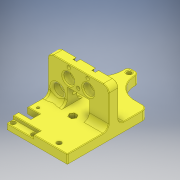
# Autodesk Inventor part: Extruder Mount cyclops mit ir probe _ rounded
Saved by Autodesk Inventor 2019 (Build 230136000, 136)
## iProperties
Created: 2016-03-27
Part Number: Extruder Mount cyclops mit ir probe _ rounded
Material: ABS Plastic
Document SubType Name: Modeling
Designer: Scott
Mass: 47.0424 g
Surface Area: 151.913 cm^2
Volume: 44.3796 cm^3
Density: 1.06 g/cm^3
Appearance: Smooth - Yellow
Author: Scott
## iProperties of the stored document Extruder Mount cyclops mit ir probe_3D-Druck.ipt
Created: 2018-12-29
Part Number: Extruder Mount cyclops mit ir probe_3D-Druck
Material: Generisch
Document SubType Name: Modeling
Designer: marc
Density: 1 g/cm^3
Appearance: Vorgabe
Author: marc
Autodesk Inventor part; units mm, degrees
ref_plane "YZ Plane" through (0, 0, 0) normal (1, 0, 0) x (0, 1, 0)
ref_plane "XZ Plane" through (0, 0, 0) normal (0, 1, 0) x (-1, 0, 0)
sketch "Sketch1" plane through (0, 0, 0) normal (0, 0, 1) x (1, 0, 0)
  line L0 (0, 0) -> (85, 0)
  line L1 (85, 0) -> (85, 83.5)
  line L2 (85, 83.5) -> (0, 83.5)
  line L3 (0, 83.5) -> (0, 0)
  dimension "d0" = 85
  dimension "d1" = 83.5
  constraints: 8 end point, 2 parallel, 1 horizontal, 1 perpendicular
  measures "d0" distance of L1.end L2.end
  measures "d1" distance of L0.end L1.end
extrude "Extrusion1" add sketch "Sketch1" along normal blind 5
sketch "Sketch10" plane through (0, 0, 5) normal (0, 0, 1) x (1, 0, 0)
  line L0 (85, 0) -> (85, 83.5) projected
  line L1 (85, 83.5) -> (0, 83.5) projected
  line L2 (0, 83.5) -> (0, 0) projected
  circle A0 centre (15.5, 75) radius 2.25 projected
  circle A1 centre (15.5, 75) radius 4
  circle A2 centre (33.5, 75) radius 4
  circle A3 centre (51.5, 75) radius 4
  circle A4 centre (69.5, 75) radius 4
  circle A5 centre (33.5, 51) radius 2.25 projected
  line L3 (0, 0) -> (85, 0) projected
  circle A6 centre (33.5, 30) radius 4
  circle A7 centre (51.5, 30) radius 4
  circle A8 centre (33.5, 6) radius 4
  circle A9 centre (51.5, 6) radius 4
  line L4 (85, 0) -> (85, 83.5) projected
  line L5 (85, 83.5) -> (0, 83.5) projected
  line L6 (0, 83.5) -> (0, 0) projected
  line L7 (0, 0) -> (85, 0) projected
  circle A10 centre (15.5, 51) radius 2.25 projected
  circle A11 centre (15.5, 51) radius 4
  circle A12 centre (33.5, 51) radius 4
  circle A13 centre (51.5, 51) radius 4
  circle A14 centre (69.5, 51) radius 4
  circle A15 centre (37.75, 40.5) radius 1.5 projected
  circle A16 centre (47.25, 40.5) radius 1.5 projected
  circle A17 centre (37.75, 40.5) radius 2.75
  circle A18 centre (47.25, 40.5) radius 2.75
  dimension "d73" = 8
  dimension "d152" = 5.5
  constraints: 14 centre point, 12 equal radius, 5 coincident
  measures "d73" diameter of A1
  measures "d152" diameter of A17
extrude "Grundplatte" add sketch "Sketch10" along normal blind 4 contours L3 L2 L1 L0 | A0 | A1 | A2 | A3 | A4 | A5 | A6 | A7 | A8 | A9 | A10 | A11 | A12 | A13 | A14 | A15 | A16 | A17 | A18
sketch "Sketch24" plane through (0, 0, 9) normal (0, 0, 1) x (1, 0, 0)
  line L0 (9.5, 63.9289) -> (9.5, 2) projected
  line L1 (75.5, 2) -> (75.5, 63.9289) projected
  line L2 (75.5, 63.9289) -> (75.5, 2) projected
  line L3 (9.5, 46.85) -> (75.5, 46.85)
  line L4 (75.5, 46.85) -> (75.5, 38.15)
  line L5 (75.5, 38.15) -> (9.5, 38.15)
  line L6 (9.5, 38.15) -> (9.5, 46.85)
  line L7 (0, 0) -> (85, 0) projected
  point P0 (11.5, 0)
  point P1 (73.5, 0)
  dimension "d173" = 8.7
  dimension "d174" = 38.15
  constraints: 8 end point, 2 parallel, 2 point on line, 1 horizontal, 1 perpendicular
  measures "d173" distance between parallel lines of L5 L3
  measures "d174" distance between parallel lines of L7 L5
extrude "Hotend_Brücke" add sketch "Sketch24" along normal blind 34
sketch "Sketch25" plane through (2, 83.5, 0) normal (0, 1, 0) x (1, 0, 0)
  line L0 (40.5, -18) -> (40.5, -43) construction
  line L1 (73.5, -43) -> (7.5, -43) construction
  line L2 (30.5, -9) -> (30.5, -24.2)
  line L3 (30.5, -24.2) -> (50.5, -24.2)
  line L4 (83, -9) -> (-2, -9) projected
  line L5 (50.5, -24.2) -> (50.5, -9)
  line L6 (50.5, -9) -> (30.5, -9)
  point P0 (-2, 0)
  point P1 (0, -9)
  dimension "d177" = 20
  dimension "d348" = 15.2
  constraints: 10 end point, 1 collinear, 1 midpoint, 1 perpendicular, 1 vertical
  measures "d177" distance of L2.end L3.end
  measures "d348" distance of L2.start L2.end
extrude "Luftdurchlass" cut sketch "Sketch25" against normal through all
sketch "Sketch39" plane through (32.5, 46.85, 24.2) normal (0, 1, 0) x (1, 0, 0)
  line L0 (0, 0) -> (0, 15.2) projected
  circle A0 centre (0, 7.6) radius 1.25
  point P0 (-32.5, 24.2)
  dimension "d263" = 2.5
  constraints: 1 centre point, 1 midpoint
  measures "d263" diameter of A0
extrude "Extrusion35" cut sketch "Sketch39" against normal blind 4
fillet "Fillet23" radius 1 1 edges at (31.25, 42.85, 16.6)
sketch "Sketch40" plane through (32.5, 46.85, 24.2) normal (0, 1, 0) x (1, 0, 0)
  line L0 (20, 15.2) -> (20, 0) projected
  line L1 (24, 7.35) -> (33, 7.35)
  line L2 (34, 8.35) -> (34, 8.6)
  line L3 (34, 8.6) -> (23, 8.6)
  line L4 (23, 8.6) -> (23, 8.35)
  arc A0 (23, 8.35) -> (24, 7.35) centre (24, 8.35) ccw
  arc A1 (33, 7.35) -> (34, 8.35) centre (33, 8.35) ccw
  line L5 (20, 0) -> (0, 0) projected
  point P0 (-32.5, 24.2)
  point P1 (23, 7.35)
  dimension "d267" = 1.25
  dimension "d268" = 3
  dimension "d269" = 14
  dimension "d270" = 1
  dimension "d332" = 8.6
  constraints: 8 end point, 4 point on circle, 4 tangent, 2 centre point, 2 parallel, 2 point on line, 1 equal radius, 1 horizontal, 1 perpendicular
  measures "d267" distance of L3.end point (23, 7.35)
  measures "d268" distance between parallel lines of L4 L0
  measures "d269" distance between parallel lines of L2 L0
  measures "d270" radius of A0
  measures "d332" distance between parallel lines of L5 L3
revolve "Revolution1" cut sketch "Sketch40" angle 180 about axis through (66.5, 46.85, 15.6) along (1, 0, 0)
sketch "Sketch45" plane through (0, 0, 9) normal (0, 0, 1) x (1, 0, 0)
  line L0 (85, 83.5) -> (0, 83.5) projected
  line L1 (75.5, 46.85) -> (75.5, 63.9289) projected
  arc A0 (76.9645, 67.4645) -> (75.5, 63.9289) centre (80.5, 63.9289) ccw projected
  line L2 (76.9645, 67.4645) -> (84.4142, 74.9142) projected
  arc A1 (84.4142, 74.9142) -> (85, 76.3284) centre (83, 76.3284) ccw projected
  line L3 (85, 0) -> (85, 83.5) projected
  arc A2 (85, 81.5) -> (83, 83.5) centre (83, 81.5) ccw projected
  line L4 (85, 83.5) -> (0, 83.5) projected
  line L5 (75.5, 63.5) -> (85, 63.5)
  line L6 (85, 63.5) -> (85, 83.5)
  line L7 (85, 83.5) -> (75.5, 83.5)
  line L8 (75.5, 83.5) -> (75.5, 63.5)
  point P0 (0, 0)
  point P1 (43, 83.5)
  point P2 (75.5, 58.85)
  point P3 (41, 83.5)
  point P4 (75.5, 56.85)
  point P5 (2, 83.5)
  dimension "d301" = 20
  constraints: 9 end point, 2 parallel, 1 collinear, 1 horizontal, 1 perpendicular, 1 point on line
  measures "d301" distance between parallel lines of L0 L5
extrude "Extrusion39" cut sketch "Sketch45" against normal through all
sketch "Sketch51" plane through (0, 0, 0) normal (0, 0, -1) x (-1, 0, 0)
  line L0 (-75.5, 46.85) -> (-75.5, 38.15) construction
  line L1 (-9.5, 38.15) -> (-9.5, 46.85) construction
  line L2 (-75.5, 42.5) -> (-9.5, 42.5) construction
  line L3 (-75.5, 83.5) -> (0, 83.5) projected
  line L4 (0, 0) -> (-85, 0) projected
  line L5 (-70, 83.5) -> (-85, 83.5)
  line L6 (-85, 83.5) -> (-85, 0)
  line L7 (-85, 0) -> (-70, 0)
  line L8 (-70, 0) -> (-70, 83.5)
  line L9 (-42.5, 100.2) -> (-42.5, -16.7) projected
  line L10 (-15, 83.5) -> (0, 83.5)
  line L11 (0, 83.5) -> (0, 0)
  line L12 (0, 0) -> (-15, 0)
  line L13 (-15, 0) -> (-15, 83.5)
  dimension "d349" = 27.5
  dimension "d350" = 27.5
  constraints: 18 end point, 4 parallel, 2 horizontal, 2 midpoint, 2 perpendicular, 2 point on line
  measures "d349" distance between parallel lines of L8 L9
  measures "d350" distance between parallel lines of L13 L9
extrude "Extrusion43" cut sketch "Sketch51" against normal through all contours L3 L8 L4 L6 L5 | L3 L11 L4 L13
sketch "Sketch52" plane through (0, 0, 0) normal (0, 0, -1) x (-1, 0, 0)
  line L0 (-15, 46.85) -> (-15, 38.15) construction
  line L1 (-70, 38.15) -> (-70, 46.85) construction
  line L2 (-42.5, 100.2) -> (-42.5, -16.7) construction
  line L3 (-70, 83.5) -> (-15, 83.5) construction
  line L4 (-70, 83.5) -> (-70, 0) construction
  line L5 (-15, 0) -> (-70, 0) construction
  line L6 (-15, 0) -> (-15, 83.5) construction
  line L7 (-70, 83.5) -> (-15, 83.5) construction
  line L8 (-15, 83.5) -> (-15, 46.85) projected
  line L9 (-70, 83.5) -> (-15, 83.5)
  line L10 (-15, 83.5) -> (-15, 65.75)
  line L11 (-15, 65.75) -> (-70, 65.75)
  line L12 (-70, 65.75) -> (-70, 83.5)
  line L13 (-70, 41.75) -> (-15, 41.75) construction
  line L14 (-15, 0) -> (-70, 0) projected
  line L15 (-15, 38.15) -> (-15, 0) projected
  line L16 (-70, 0) -> (-15, 0)
  line L17 (-15, 0) -> (-15, 0.75)
  line L18 (-15, 0.75) -> (-70, 0.75)
  line L19 (-70, 0.75) -> (-70, 0)
  point P0 (0, 0)
  dimension "d353" = 24
  dimension "d373" = 65
  constraints: 18 end point, 4 parallel, 2 horizontal, 2 midpoint, 2 perpendicular, 2 point on line
  measures "d353" distance between parallel lines of L11 L13
  measures "d373" distance between parallel lines of L18 L11
extrude "Extrusion44" cut sketch "Sketch52" against normal through all
sketch "Sketch55" plane through (0, 0, 0) normal (0, 0, -1) x (-1, 0, 0)
  line L0 (-15, 0.75) -> (-15, 65.75) projected
  line L1 (-15, 65.75) -> (-15, 46.85) projected
  line L2 (-15, 38.15) -> (-15, 0.75) projected
  line L3 (-26, 46.75) -> (-15, 46.75)
  line L4 (-15, 46.75) -> (-15, 11.75)
  line L5 (-15, 11.75) -> (-26, 11.75)
  line L6 (-26, 11.75) -> (-26, 46.75)
  point P0 (0, 0)
  dimension "d374" = 19
  dimension "d375" = 11
  dimension "d376" = 11
  constraints: 8 end point, 2 parallel, 1 horizontal, 1 perpendicular, 1 point on line
  measures "d374" distance from line of L0.end L3
  measures "d375" distance from line of L0.start L5
  measures "d376" distance of L3.start L3.end
extrude "Extrusion45" cut sketch "Sketch55" against normal blind 3.5
sketch "Sketch56" plane through (0, 0, 0) normal (0, 0, -1) x (-1, 0, 0)
  line L0 (-70, 65.75) -> (-15, 65.75) construction
  line L1 (-42.5, 65.75) -> (-42.5, 0.75) construction
  line L2 (-15, 0.75) -> (-70, 0.75) construction
  line L3 (-54.5, 45.25) -> (-30.5, 45.25) construction
  line L4 (-30.5, 45.25) -> (-30.5, 21.25) construction
  line L5 (-30.5, 21.25) -> (-54.5, 21.25) construction
  line L6 (-54.5, 21.25) -> (-54.5, 45.25) construction
  line L7 (-30.5, 45.25) -> (-54.5, 21.25) construction
  line L8 (-54.5, 45.25) -> (-30.5, 21.25) construction
  point P0 (0, 0)
  point P1 (-42.5, 33.25)
  dimension "d379" = 24
  dimension "d380" = 24
  constraints: 14 end point, 4 midpoint, 3 coincident, 2 parallel, 1 horizontal, 1 perpendicular, 1 point on line
  measures "d379" distance of L3.start L3.end
  measures "d380" distance of L3.end L4.end
hole "Hole14" at (42.5, 33.25, 0) at (54.5, 45.25, 0) at (54.5, 21.25, 0) at (30.5, 21.25, 0) at (30.5, 45.25, 0) direction (0, 0, 1) diameter 3 depth 8
sketch "Sketch57" plane through (0, 0, 0) normal (0, 0, -1) x (-1, 0, 0)
  circle A0 centre (-42.5, 33.25) radius 1.5 projected
  point P0 (0, 0)
  constraints: 1 coincident
hole "Hole15" at (42.5, 33.25, 0) direction (0, 0, 1) diameter 4.2 end through all
ref_plane "Work Plane14" through (42.5, 37.25, 33.75) normal (1, 0, 0) x (0, -1, 0)
sketch "Sketch58" plane through (0, 0, 3.5) normal (0, 0, -1) x (-1, 0, 0)
  circle A0 centre (-42.5, 33.25) radius 2.1 construction
  line L0 (-42.5, 33.25) -> (-7.5484, 33.25) construction
  line L1 (-15, 46.75) -> (-15, 11.75) construction
  line L2 (-26, 46.75) -> (-15, 46.75) construction
  line L3 (-26, 11.75) -> (-26, 46.75) construction
  line L4 (-15, 11.75) -> (-26, 11.75) construction
  line L5 (-25.2, 39.25) -> (-15.8, 39.25)
  line L6 (-15.8, 39.25) -> (-15.8, 27.25)
  line L7 (-15.8, 27.25) -> (-25.2, 27.25)
  line L8 (-25.2, 27.25) -> (-25.2, 39.25)
  point P0 (0, 0)
  dimension "d396" = 6
  dimension "d397" = 6
  dimension "d398" = 0.8
  dimension "d399" = 0.8
  constraints: 10 end point, 2 horizontal, 2 parallel, 1 perpendicular
  measures "d396" distance between parallel lines of L0 L5
  measures "d397" distance between parallel lines of L0 L7
  measures "d398" distance between parallel lines of L1 L6
  measures "d399" distance between parallel lines of L3 L8
extrude "Extrusion46" cut sketch "Sketch58" against normal blind 1.5
sketch "Sketch59" plane through (0, 0, 3.5) normal (0, 0, -1) x (-1, 0, 0)
  circle A0 centre (-42.5, 33.25) radius 2.1 construction
  line L0 (-42.5, 33.25) -> (-9.4661, 33.25) construction
  line L1 (-20.5, 50.9301) -> (-20.5, 7.336) construction
  line L2 (-15, 46.75) -> (-15, 11.75) projected
  point P0 (0, 0)
  point P1 (-20.5, 42.775)
  point P2 (-20.5, 23.725)
  dimension "d402" = 5.5
  dimension "d403" = 9.525
  dimension "d404" = 9.525
  constraints: 4 end point, 2 point on line, 1 horizontal, 1 vertical
  measures "d402" distance between parallel lines of L2 L1
  measures "d403" distance from line of L0 point (-20.5, 42.775)
  measures "d404" distance from line of L0 point (-20.5, 23.725)
hole "Hole16" at (20.5, 42.775, 3.5) at (20.5, 23.725, 3.5) direction (0, 0, 1) diameter 2.5 depth 8
sketch "Skizze69" plane through (32.5, 46.85, 24.2) normal (0, 1, 0) x (1, 0, 0)
  line L0 (-17.5, 15.2) -> (-17.5, -18.8) projected
  line L1 (37.5, -18.8) -> (37.5, 15.2) projected
  line L2 (37.5, 15.2) -> (-17.5, 15.2) projected
  line L3 (37.5, -18.8) -> (-17.5, -18.8) projected
  line L4 (20, 0) -> (0, 0) projected
  point P0 (-32.5, 24.2)
  point P1 (10, -4)
  point P2 (19, -7)
  point P3 (18.5, -16)
  point P4 (1.5, -16)
  point P5 (1, -7)
  dimension "d487" = 55
  dimension "d488" = 34
  dimension "d489" = 27.5
  dimension "d490" = 4
  dimension "d491" = 7
  dimension "d492" = 9
  dimension "d493" = 16
  dimension "d494" = 8.5
  dimension "d495" = 8.5
  dimension "d496" = 9
  constraints: 2 horizontal alignment
  measures "d487" distance between parallel lines of L0 L1
  measures "d488" distance between parallel lines of L2 L3
  measures "d489" distance from line of L0 point (10, -4)
  measures "d490" distance from line of L4 point (10, -4)
  measures "d491" distance from line of L4 point (19, -7)
  measures "d492" horizontal distance of point (10, -4) point (19, -7)
  measures "d493" distance from line of L4 point (18.5, -16)
  measures "d494" horizontal distance of point (10, -4) point (18.5, -16)
  measures "d495" horizontal distance of point (10, -4) point (1.5, -16)
  measures "d496" horizontal distance of point (10, -4) point (1, -7)
hole "Bohrung20" at (51, 46.85, 40.2) at (34, 46.85, 40.2) at (42.5, 46.85, 28.2) direction (0, -1, 0) diameter 3.2 end through all counterbore diameter 6.5 counterbore depth 3.4 clearance for "Inbusschraube ISO 4762" size "M3" standard "ISO"
hole "Bohrung21" at (51.5, 46.85, 31.2) at (33.5, 46.85, 31.2) direction (0, -1, 0) diameter 10 end through all
sketch "Skizze70" plane through (52.5, 46.85, 24.2) normal (0, 1, 0) x (1, 0, 0)
  line L0 (-37.5, 15.2) -> (-37.5, -18.8) projected
  line L1 (-20, 0) -> (-20, 6.35) projected
  line L2 (17.5, 15.2) -> (-37.5, 15.2) projected
  point P0 (-52.5, 24.2)
  point P1 (-28.75, 7.2)
  dimension "d511" = 8.75
  dimension "d512" = 17.5
  dimension "d513" = 8
  measures "d511" distance from line of L0 point (-28.75, 7.2)
  measures "d512" distance between parallel lines of L0 L1
  measures "d513" distance from line of L2 point (-28.75, 7.2)
hole "Bohrung22" at (23.75, 46.85, 17) direction (0, -1, 0) diameter 10 end through all
sketch "Skizze71" plane through (15, 65.75, 0) normal (0, 1, 0) x (1, 0, 0)
  line L0 (55, -9) -> (0, -9) projected
  line L1 (55, 0) -> (55, -9) projected
  line L2 (0, 0) -> (55, 0) projected
  line L3 (0, -9) -> (0, 0) projected
  point P0 (-15, 0)
extrude "Extrusion53" add sketch "Skizze71" along normal blind 8
sketch "Skizze72" plane through (0, 0, 9) normal (0, 0, 1) x (1, 0, 0)
  line L0 (15, 73.75) -> (15, 46.85) projected
  line L1 (15, 0.75) -> (70, 0.75) projected
  line L2 (15, 73.75) -> (70, 73.75) projected
  point P0 (0, 0)
  point P1 (24, 69.75)
  point P2 (19, 69.75)
  dimension "d523" = 5
  dimension "d527" = 4
  dimension "d533" = 4
  constraints: 1 horizontal alignment
  measures "d523" distance of point (19, 69.75) point (24, 69.75)
  measures "d527" distance from line of L0 point (19, 69.75)
  measures "d533" distance from line of L2 point (19, 69.75)
hole "Bohrung23" at (24, 69.75, 9) at (19, 69.75, 9) direction (0, 0, -1) diameter 4 end through all
sketch "Skizze74" plane through (0, 0, 9) normal (0, 0, 1) x (1, 0, 0)
  line L0 (42.5, 11.75) -> (26, 11.75) projected
  line L1 (15, 38.15) -> (15, 46.85) projected
  line L2 (70, 0.75) -> (70, 38.15) projected
  point P0 (0, 0)
  point P1 (59, 11.75)
  point P2 (15, 18.75)
  point P3 (70, 18.75)
  point P4 (68.5, 11.75)
  dimension "d541" = 27.5
  dimension "d542" = 27.5
  dimension "d543" = 55
  constraints: 1 end point
  measures "d541" distance from line of L1 L0.start
  measures "d542" distance from line of L2 L0.start
  measures "d543" distance between parallel lines of L2 L1
sketch "Skizze73" plane through (0, 0, 9) normal (0, 0, 1) x (1, 0, 0)
  line L0 (42.5, 88.5) -> (42.5, -14.75) projected
  line L1 (15, 0.75) -> (70, 0.75) projected
  line L2 (70, 0.75) -> (70, 11.45) projected
  line L3 (15, 11.45) -> (15, 0.75) projected
  point P0 (0, 0)
  point P1 (18, 3.75)
  point P2 (36.41, 3.75)
  point P3 (57.5, 5.75)
  dimension "d544" = 15
  dimension "d546" = 5
  dimension "d547" = 3
  dimension "d548" = 18.41
  dimension "d550" = 3
  constraints: 1 horizontal alignment
  measures "d544" distance from line of L0 point (57.5, 5.75)
  measures "d546" distance from line of L1 point (57.5, 5.75)
  measures "d547" distance from line of L1 point (36.41, 3.75)
  measures "d548" distance of point (36.41, 3.75) point (18, 3.75)
  measures "d550" distance from line of L3 point (18, 3.75)
sketch "Skizze75" plane through (0, 0, 9) normal (0, 0, 1) x (1, 0, 0)
  line L0 (15, 0.75) -> (70, 0.75) projected
  line L1 (15, 0.75) -> (39.5, 0.75)
  line L2 (39.5, 0.75) -> (39.5, 6.75)
  line L3 (39.5, 6.75) -> (15, 6.75)
  line L4 (15, 6.75) -> (15, 0.75)
  point P0 (0, 0)
  dimension "d551" = 24.5
  dimension "d552" = 6
  constraints: 8 end point, 2 parallel, 1 horizontal, 1 perpendicular
  measures "d551" distance of L2.end L3.end
  measures "d552" distance of L1.end L2.end
extrude "Extrusion54" cut sketch "Skizze75" against normal blind 3
hole "Bohrung24" at (18, 3.75, 9) at (36.41, 3.75, 9) at (57.5, 5.75, 9) direction (0, 0, -1) diameter 4.2 depth 8
fillet "Rundung34" radius 2 2 edges at (23.75, 46.85, 12) (23.75, 38.15, 12)
fillet "Rundung35" radius 2 2 edges at (33.5, 46.85, 26.2) (51.5, 46.85, 26.2)
fillet "Rundung36" radius 1 2 edges at (33.5, 38.15, 26.2) (51.5, 38.15, 26.2)
fillet "Rundung37" radius 5 2 edges at (15, 42.5, 43) (70, 42.5, 43)
fillet "Rundung38" radius 5 4 edges at (23.75, 38.15, 9) (61.25, 38.15, 9) (23.75, 46.85, 9) (61.25, 46.85, 9)
fillet "Rundung39" radius 5 2 edges at (15, 73.75, 4.5) (70, 73.75, 4.5)
fillet "Rundung40" radius 1 2 edges at (15, 0.75, 3) (70, 0.75, 4.5)
sketch "Skizze76" plane through (0, 0, 3.5) normal (0, 0, -1) x (-1, 0, 0)
  line L0 (-26, 11.75) -> (-26, 46.75) projected
  line L1 (-15, 11.75) -> (-26, 11.75)
  line L2 (-26, 11.75) -> (-26, 19.75)
  line L3 (-26, 19.75) -> (-15, 19.75)
  line L4 (-15, 19.75) -> (-15, 11.75)
  line L5 (-15, 46.75) -> (-15, 11.75) projected
  point P0 (0, 0)
  dimension "d576" = 8
  dimension "d577" = 11
  dimension "d578" = 11
  constraints: 8 end point, 2 parallel, 2 point on line, 1 horizontal, 1 perpendicular
  measures "d576" distance of L3.end L1.start
  measures "d577" distance of L2.end L3.end
  measures "d578" distance between parallel lines of L0 L5
extrude "Extrusion55" cut sketch "Skizze76" against normal blind 10
sketch "Skizze77" plane through (0, 0, 9) normal (0, 0, 1) x (1, 0, 0)
  circle A0 centre (42.5, 33.25) radius 1.5 projected
  line L0 (15, 19.75) -> (26, 19.75) projected
  line L1 (26, 19.75) -> (26, 11.75) projected
  line L2 (26, 11.75) -> (15, 11.75) projected
  line L3 (15, 11.75) -> (15, 6.75) projected
  line L4 (15, 6.75) -> (39.5, 6.75) projected
  line L5 (39.5, 6.75) -> (39.5, 0.75) projected
  line L6 (39.5, 0.75) -> (69, 0.75) projected
  arc A1 (69, 0.75) -> (70, 1.75) centre (69, 1.75) ccw projected
  line L7 (70, 1.75) -> (70, 33.15) projected
  line L8 (52.5, 33.15) -> (70, 33.15) projected
  line L9 (52.5, 51.85) -> (52.5, 33.15) projected
  line L10 (70, 51.85) -> (52.5, 51.85) projected
  line L11 (70, 51.85) -> (70, 68.75) projected
  arc A2 (70, 68.75) -> (65, 73.75) centre (65, 68.75) ccw projected
  line L12 (20, 73.75) -> (65, 73.75) projected
  arc A3 (20, 73.75) -> (15, 68.75) centre (20, 68.75) ccw projected
  line L13 (15, 68.75) -> (15, 51.85) projected
  line L14 (17.4254, 51.85) -> (15, 51.85) projected
  line L15 (32.5, 51.85) -> (30.0746, 51.85) projected
  line L16 (32.5, 51.85) -> (32.5, 33.15) projected
  line L17 (30.0746, 33.15) -> (32.5, 33.15) projected
  line L18 (15, 33.15) -> (17.4254, 33.15) projected
  line L19 (15, 33.15) -> (15, 19.75) projected
  circle A4 centre (20.5, 23.725) radius 1.25 projected
  circle A5 centre (19, 69.75) radius 2 projected
  line L20 (44.0877, 36) -> (45.6754, 33.25)
  line L21 (45.6754, 33.25) -> (44.0877, 30.5)
  line L22 (44.0877, 30.5) -> (40.9123, 30.5)
  line L23 (40.9123, 30.5) -> (39.3246, 33.25)
  line L24 (39.3246, 33.25) -> (40.9123, 36)
  line L25 (40.9123, 36) -> (44.0877, 36)
  line L26 (20, 38.15) -> (65, 38.15) projected
  point P0 (0, 0)
  dimension "d581" = 5.5
  constraints: 12 end point, 2 horizontal alignment, 1 coincident, 1 parallel, 13 other
  measures "d581" distance between parallel lines of L22 L25
extrude "Extrusion56" cut sketch "Skizze77" against normal blind 4 contours L20 L21 L22 L23 L24 L25
sketch "Skizze78" plane through (15, 73.75, 0) normal (0, 1, 0) x (1, 0, 0)
  line L0 (50, 0) -> (5, 0) projected
  line L1 (5, -9) -> (50, -9) projected
  line L2 (14, 0) -> (24, 0)
  line L3 (24, 0) -> (24, -9)
  line L4 (24, -9) -> (14, -9)
  line L5 (14, -9) -> (14, 0)
  line L6 (5, -9) -> (5, 0) projected
  point P0 (-15, 0)
  dimension "d584" = 10
  dimension "d585" = 9
  constraints: 8 end point, 2 parallel, 2 point on line, 1 horizontal, 1 perpendicular
  measures "d584" distance between parallel lines of L5 L3
  measures "d585" distance between parallel lines of L6 L5
extrude "Extrusion57" add sketch "Skizze78" along normal blind 23 contours L3 L1 L5 L0
sketch "Skizze79" plane through (0, 0, 9) normal (0, 0, 1) x (1, 0, 0)
  line L0 (39, 73.75) -> (39, 96.75) projected
  line L1 (29, 73.75) -> (29, 96.75) projected
  line L2 (29, 96.75) -> (39, 96.75) projected
  point P0 (0, 0)
  point P1 (34, 92.75)
  dimension "d588" = 10
  dimension "d589" = 4
  dimension "d590" = 5
  measures "d588" distance between parallel lines of L0 L1
  measures "d589" distance from line of L2 point (34, 92.75)
  measures "d590" distance from line of L0 point (34, 92.75)
hole "Bohrung25" at (34, 92.75, 9) direction (0, 0, -1) diameter 4 end through all
sketch "Skizze80" plane through (0, 0, 0) normal (0, 0, -1) x (-1, 0, 0)
  circle A0 centre (-34, 92.75) radius 2 projected
  line L0 (-35.5877, 90) -> (-37.1754, 92.75)
  line L1 (-37.1754, 92.75) -> (-35.5877, 95.5)
  line L2 (-35.5877, 95.5) -> (-32.4123, 95.5)
  line L3 (-32.4123, 95.5) -> (-30.8246, 92.75)
  line L4 (-30.8246, 92.75) -> (-32.4123, 90)
  line L5 (-32.4123, 90) -> (-35.5877, 90)
  line L6 (-39, 96.75) -> (-29, 96.75) projected
  point P0 (0, 0)
  dimension "d598" = 5.5
  constraints: 12 end point, 1 coincident, 1 parallel, 13 other
  measures "d598" distance between parallel lines of L2 L5
extrude "Extrusion59" cut sketch "Skizze80" against normal blind 4
fillet "Rundung42" radius 3.5 2 edges at (39, 96.75, 4.5) (29, 96.75, 4.5)
fillet "Rundung43" radius 19.5 1 edges at (39, 73.75, 4.5)
fillet "Rundung44" radius 19.5 1 edges at (29, 73.75, 4.5)
chamfer "Fase6" distance 1 angle 45 15 edges at (25.9805, 80.4628, 0) (15.7742, 71.4226, 0) (15, 57.75, 0) (29, 92.068, 0) (30.0251, 95.7249, 0) (34, 96.75, 0) (37.9749, 95.7249, 0) (44.7114, 79.4614, 0) (61.75, 73.75, 0) (68.5355, 72.2855, 0) (70, 35.25, 0) (69.7071, 1.0429, 0) (42.5, 0.75, 0) (15.2929, 1.0429, 0) (15, 6.75, 0)
chamfer "Fase7" distance 1 angle 45 5 edges at (30.5, 43.75, 0) (30.5, 19.75, 0) (42.5, 31.15, 0) (54.5, 19.75, 0) (54.5, 43.75, 0)
fillet "Rundung45" radius 0.2 6 edges at (31.6184, 91.375, 0) (31.6184, 94.125, 0) (34, 95.5, 0) (36.3816, 94.125, 0) (36.3816, 91.375, 0) (34, 90, 0)
fillet "Rundung46" radius 0.2 6 edges at (42.5, 36, 9) (44.8816, 34.625, 9) (44.8816, 31.875, 9) (42.5, 30.5, 9) (40.1184, 31.875, 9) (40.1184, 34.625, 9)
fillet "Rundung47" radius 0.8 1 edges at (34, 94.75, 9)
fillet "Rundung48" radius 0.5 4 edges at (24, 71.75, 9) (19, 71.75, 9) (19, 71.75, 0) (24, 71.75, 0)
fillet "Rundung49" radius 0.5 39 edges at (15.7742, 71.4226, 9) (15, 60.3, 9) (15, 48.3145, 10.4645) (15, 46.85, 26) (16.4645, 46.85, 41.5355) (26.175, 46.85, 43) (29, 92.068, 9) (30.0251, 95.7249, 9) (34, 96.75, 9) (37.9749, 95.7249, 9) (44.7114, 79.4614, 9) (61.75, 73.75, 9) (68.5355, 72.2855, 9) (70, 60.3, 9) (70, 48.3145, 10.4645) (70, 46.85, 26) (68.5355, 46.85, 41.5355) (58.825, 46.85, 43) (25.9805, 80.4628, 9) (70, 36.6855, 10.4645) (70, 38.15, 26) (68.5355, 38.15, 41.5355) (42.5, 38.15, 43) (16.4645, 38.15, 41.5355) (15, 38.15, 26) (15, 36.6855, 10.4645) (15, 26.45, 9) (69.7071, 1.0429, 9) (54.25, 0.75, 9) (70, 17.45, 9) (26, 15.75, 9) (20.5, 19.75, 9) (20.5, 11.75, 9) (15, 9.25, 9) (27.25, 6.75, 9) (15.2929, 1.0429, 6) (27.75, 0.75, 6) (15, 4.25, 6) (39.5, 3.75, 9)
body "Solid1"
